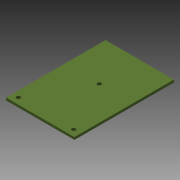
# Autodesk Inventor part: Testplatine
Saved by Autodesk Inventor 2015 (Build 190159000, 159)
## iProperties
Created: 2015-03-02
Part Number: Testplatine
Material: Generisch
Document SubType Name: Modeling
Designer: TowerSebi
Density: 1 g/cm^3
Appearance: Olivgrün
Author: TowerSebi
Autodesk Inventor part; units mm, degrees
ref_plane "YZ Plane" through (0, 0, 0) normal (1, 0, 0) x (0, 1, 0)
ref_plane "XZ Plane" through (0, 0, 0) normal (0, 1, 0) x (-1, 0, 0)
ref_plane "XY Plane" through (0, 0, 0) normal (0, 0, 1) x (1, 0, 0)
sketch "Skizze1" plane through (0, 0, 0) normal (0, 0, 1) x (1, 0, 0)
  line L0 (0, 0) -> (55, 0)
  line L1 (55, 0) -> (55, 80)
  line L2 (55, 80) -> (0, 80)
  line L3 (0, 80) -> (0, 0)
  circle A0 centre (5, 5) radius 1.6
  circle A1 centre (49.5, 5) radius 1.6
  circle A2 centre (28, 47) radius 1.6
  dimension "d0" = 80
  dimension "d1" = 55
  dimension "d2" = 3.2
  dimension "d3" = 3.2
  dimension "d4" = 3.2
  dimension "d5" = 5
  dimension "d6" = 5
  dimension "d7" = 49.5
  dimension "d8" = 5
  dimension "d9" = 47
  dimension "d10" = 28
  constraints: 8 end point, 3 centre point, 2 parallel, 1 horizontal, 1 perpendicular
  measures "d0" distance of L2.end L0.start
  measures "d1" distance of L0.start L0.end
  measures "d2" diameter of A2
  measures "d3" diameter of A1
  measures "d4" diameter of A0
  measures "d5" distance from line of A0.centre L3
  measures "d6" distance from line of L0 A0.centre
  measures "d7" distance from line of L3 A1.centre
  measures "d8" distance from line of L0 A1.centre
  measures "d9" distance from line of L0 A2.centre
  measures "d10" distance from line of L3 A2.centre
extrude "Extrusion1" add sketch "Skizze1" along normal blind 2
